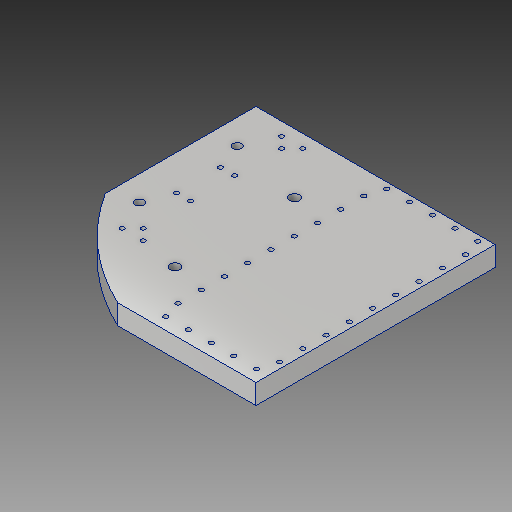
# Autodesk Inventor part: Base Plate Mk 2
Saved by Autodesk Inventor 2017 (Build 210142000, 142)
## iProperties
Created: 2016-12-06
Part Number: Base Plate Mk 2
Material: Aluminum 6061
Document SubType Name: Modeling
Designer: qupec
Density: 2.7 g/cm^3
Appearance: Aluminum - Flat
Mass: 732.131 g
Surface Area: 558.67 cm^2
Volume: 271.16 cm^3
Author: qupec
Autodesk Inventor part; units mm, degrees
ref_plane "YZ Plane" through (0, 0, 0) normal (1, 0, 0) x (0, 1, 0)
ref_plane "XZ Plane" through (0, 0, 0) normal (0, 1, 0) x (-1, 0, 0)
ref_plane "XY Plane" through (0, 0, 0) normal (0, 0, 1) x (1, 0, 0)
sketch "Sketch1" plane through (0, 0, 0) normal (0, 1, 0) x (-1, 0, 0)
  line L0 (76.2, 76.2) -> (-76.2, 76.2)
  line L1 (-76.2, 76.2) -> (-76.2, -76.2)
  line L2 (-76.2, -76.2) -> (76.2, -76.2)
  line L3 (76.2, -76.2) -> (76.2, 76.2)
  point P0 (0, 0)
  dimension "d0" = 152.4
  dimension "d1" = 152.4
  dimension "d2" = 76.2
  dimension "d3" = 76.2
  constraints: 8 end point, 2 parallel, 1 horizontal, 1 perpendicular
  measures "d0" distance of L2.end L0.start
  measures "d1" distance of L0.start L0.end
  measures "d2" distance from line of point (0, 0) L1
  measures "d3" distance from line of point (0, 0) L0
extrude "Extrusion1" add sketch "Sketch1" along normal blind 12.7
sketch "Sketch4" plane through (0, 12.7, 0) normal (0, 1, 0) x (1, 0, 0)
  circle A0 centre (69.85, 69.85) radius 3.175
  circle A1 centre (69.85, -69.85) radius 3.175
  circle A2 centre (-67.31, -52.07) radius 3.175
  line L0 (76.2, 76.2) -> (-76.2, 76.2) projected
  line L1 (76.2, -76.2) -> (76.2, 76.2) projected
  line L2 (-76.2, -76.2) -> (76.2, -76.2) projected
  line L3 (-76.2, 76.2) -> (-76.2, -76.2) projected
  circle A3 centre (-67.31, 52.07) radius 3.175
  point P0 (0, 0)
  dimension "d20" = 6.35
  dimension "d21" = 6.35
  dimension "d22" = 6.35
  dimension "d23" = 6.35
  dimension "d24" = 6.35
  dimension "d25" = 6.35
  dimension "d26" = 6.35
  dimension "d27" = 24.13
  dimension "d28" = 8.89
  dimension "d32" = 6.35
  dimension "d33" = 24.13
  dimension "d34" = 8.89
  constraints: 4 centre point
  measures "d20" diameter of A2
  measures "d21" diameter of A1
  measures "d22" diameter of A0
  measures "d23" distance from line of L0 A0.centre
  measures "d24" distance from line of L1 A0.centre
  measures "d25" distance from line of L1 A1.centre
  measures "d26" distance from line of L2 A1.centre
  measures "d27" distance from line of L2 A2.centre
  measures "d28" distance from line of L3 A2.centre
  measures "d32" diameter of A3
  measures "d33" distance from line of L0 A3.centre
  measures "d34" distance from line of L3 A3.centre
extrude "Extrusion6" [suppressed]
fillet "Fillet1" [suppressed]
sketch "Sketch7" plane through (0, 12.7, 0) normal (0, 1, 0) x (1, 0, 0)
  arc A0 (-76.2, -19.8745) -> (-11.9351, -76.2) centre (52.3545, 61.976) ccw
  line L0 (76.2, 76.2) -> (-76.2, 76.2) projected
  line L1 (76.2, -76.2) -> (76.2, 76.2) projected
  line L2 (-76.2, 76.2) -> (-76.2, -76.2) projected
  line L3 (-76.2, -76.2) -> (76.2, -76.2) projected
  line L4 (-76.2, 76.2) -> (-76.2, -76.2) projected
  arc A1 (-11.9351, -76.2) -> (-76.2, -19.8745) centre (52.3545, 61.976) ccw
  point P0 (0, 0)
  point P1 (76.2, -60.325)
  point P2 (73.025, -60.325)
  point P3 (73.025, 63.5)
  point P4 (73.025, 60.325)
  point P5 (-73.025, 63.5)
  point P6 (76.2, 60.325)
  point P7 (73.025, -63.5)
  point P8 (-76.2, 60.325)
  point P9 (-74.6455, -22.2663)
  dimension "d46" = 304.8
  dimension "d47" = 14.224
  dimension "d48" = 23.8455
  constraints: 5 point on circle, 2 centre point, 1 point on line, 3 other
  measures "d46" diameter of A0
  measures "d48" distance from line of L1 A0.centre
sketch "Sketch8" plane through (0, 12.7, 0) normal (0, 1, 0) x (1, 0, 0)
  circle A0 centre (-38.0726, -33.782) radius 1.4224 projected
  circle A1 centre (-44.8036, -27.051) radius 1.4224 projected
  circle A2 centre (-51.5346, -33.782) radius 1.4224 projected
  circle A3 centre (-51.5346, 67.818) radius 1.4224 projected
  circle A4 centre (-44.8036, 61.087) radius 1.4224 projected
  circle A5 centre (-38.0726, 67.818) radius 1.4224 projected
  circle A6 centre (-53.876, 3.1912) radius 1.4224 projected
  circle A7 centre (-53.876, 3.1912) radius 1.4224 projected
  circle A8 centre (-44.856, 3.1912) radius 1.4224 projected
  line L0 (-40.346, 0.6734) -> (-58.386, 0.6734) projected
  line L1 (-40.346, 5.7089) -> (-40.346, 0.6734) projected
  line L2 (-40.346, 5.7089) -> (-58.386, 5.7089) projected
  line L3 (-58.386, 0.6734) -> (-58.386, 5.7089) projected
  circle A9 centre (-53.876, 31.1756) radius 1.4224 projected
  circle A10 centre (-44.856, 31.1756) radius 1.4224 projected
  line L4 (-40.346, 28.6579) -> (-58.386, 28.6579) projected
  line L5 (-40.346, 33.6934) -> (-40.346, 28.6579) projected
  line L6 (-40.346, 33.6934) -> (-58.386, 33.6934) projected
  line L7 (-58.386, 28.6579) -> (-58.386, 33.6934) projected
  circle A11 centre (2.54, -39.6875) radius 3.175 construction
  circle A12 centre (2.54, 12.7127) radius 3.175 construction
  circle A13 centre (2.54, 65.1129) radius 3.175 construction
  circle A14 centre (68.58, 65.1129) radius 3.175 construction
  circle A15 centre (68.58, 12.7127) radius 3.175 construction
  circle A16 centre (68.58, -39.6875) radius 3.175 construction
extrude "Extrusion9" cut sketch "Sketch8" against normal through all contours A0 | A1 | A2 | A3 | A4 | A5 | A6 | A8 | A9 | A10
extrude "Extrusion11" cut sketch "Sketch7" against normal through all contours A0 L3 L2
sketch "Sketch10" plane through (0, 12.7, 0) normal (0, 1, 0) x (1, 0, 0)
  circle A0 centre (68.961, 72.39) radius 1.4732 projected
  arc A1 (-76.2, -19.8745) -> (-11.9351, -76.2) centre (52.3545, 61.976) ccw projected
  line L0 (-11.9351, -76.2) -> (76.2, -76.2) projected
  line L1 (76.2, -76.2) -> (76.2, 76.2) projected
  line L2 (76.2, 76.2) -> (-76.2, 76.2) projected
  line L3 (-76.2, 76.2) -> (-76.2, -19.8745) projected
  circle A2 centre (-53.876, 31.1756) radius 1.4224 projected
  circle A3 centre (-53.876, 3.1912) radius 1.4224 projected
  circle A4 centre (-44.8036, 61.087) radius 1.4224 projected
  circle A5 centre (-51.5346, -33.782) radius 1.4224 projected
  circle A6 centre (-38.0726, -33.782) radius 1.4224 projected
  circle A7 centre (-44.8036, -27.051) radius 1.4224 projected
  circle A8 centre (-51.5346, 67.818) radius 1.4224 projected
  circle A9 centre (-38.0726, 67.818) radius 1.4224 projected
  circle A10 centre (-44.856, 3.1912) radius 1.4224 projected
  circle A11 centre (-44.856, 31.1756) radius 1.4224 projected
  circle A12 centre (40.005, 72.39) radius 1.4732 projected
  circle A13 centre (54.483, 72.39) radius 1.4732 projected
  circle A14 centre (25.527, 72.39) radius 1.4732 projected
  circle A15 centre (11.049, 72.39) radius 1.4732 projected
  circle A16 centre (68.961, -68.58) radius 1.4732 projected
  circle A17 centre (54.483, -68.58) radius 1.4732 projected
  circle A18 centre (40.005, -68.58) radius 1.4732 projected
  circle A19 centre (25.527, -68.58) radius 1.4732 projected
  circle A20 centre (11.049, -68.58) radius 1.4732 projected
  point P0 (0, 0)
extrude "Extrusion13" cut sketch "Sketch10" against normal through all contours A0 | A12 | A13 | A14 | A15 | A16 | A17 | A18 | A19 | A20
sketch "Sketch11" plane through (0, 12.7, 0) normal (0, 1, 0) x (1, 0, 0)
  circle A0 centre (25.527, 72.39) radius 1.4732 projected
  circle A1 centre (54.483, 72.39) radius 1.4732 projected
  circle A2 centre (68.961, -68.58) radius 1.4732 projected
  circle A3 centre (40.005, -68.58) radius 1.4732 projected
  circle A4 centre (11.049, -68.58) radius 1.4732 projected
  circle A5 centre (7.62, -42.545) radius 1.4732 projected
  circle A6 centre (7.62, -12.9117) radius 1.4732 projected
  circle A7 centre (7.62, 16.7217) radius 1.4732 projected
  circle A8 centre (7.62, 46.355) radius 1.4732 projected
  circle A9 centre (72.39, 61.1717) radius 1.4732 projected
  circle A10 centre (72.39, 31.5383) radius 1.4732 projected
  circle A11 centre (72.39, 1.905) radius 1.4732 projected
  circle A12 centre (72.39, -27.7283) radius 1.4732 projected
  circle A13 centre (72.39, -57.3617) radius 1.4732 projected
  circle A14 centre (72.39, -42.545) radius 1.4732 projected
  circle A15 centre (72.39, -12.9117) radius 1.4732 projected
  circle A16 centre (72.39, 16.7217) radius 1.4732 projected
  circle A17 centre (72.39, 46.355) radius 1.4732 projected
  circle A18 centre (7.62, 61.1717) radius 1.4732 projected
  circle A19 centre (7.62, 31.5383) radius 1.4732 projected
  circle A20 centre (7.62, 1.905) radius 1.4732 projected
  circle A21 centre (7.62, -27.7283) radius 1.4732 projected
  circle A22 centre (7.62, -57.3617) radius 1.4732 projected
  circle A23 centre (25.527, -68.58) radius 1.4732 projected
  circle A24 centre (54.483, -68.58) radius 1.4732 projected
  circle A25 centre (68.961, 72.39) radius 1.4732 projected
  circle A26 centre (40.005, 72.39) radius 1.4732 projected
  circle A27 centre (11.049, 72.39) radius 1.4732 projected
  line L0 (6.985, -72.39) -> (73.025, -72.39) projected
  line L1 (76.2, -69.215) -> (76.2, 73.025) projected
  line L2 (73.025, 76.2) -> (6.985, 76.2) projected
  line L3 (3.81, 73.025) -> (3.81, -69.215) projected
  arc A28 (65.405, 62.23) -> (62.23, 65.405) centre (62.23, 62.23) ccw projected
  line L4 (65.405, -58.42) -> (65.405, 62.23) projected
  arc A29 (62.23, -61.595) -> (65.405, -58.42) centre (62.23, -58.42) ccw projected
  line L5 (17.78, -61.595) -> (62.23, -61.595) projected
  arc A30 (14.605, -58.42) -> (17.78, -61.595) centre (17.78, -58.42) ccw projected
  line L6 (14.605, 62.23) -> (14.605, -58.42) projected
  arc A31 (17.78, 65.405) -> (14.605, 62.23) centre (17.78, 62.23) ccw projected
  line L7 (62.23, 65.405) -> (17.78, 65.405) projected
  arc A32 (76.2, 73.025) -> (73.025, 76.2) centre (73.025, 73.025) ccw projected
  arc A33 (6.985, 76.2) -> (3.81, 73.025) centre (6.985, 73.025) ccw projected
  arc A34 (3.81, -69.215) -> (6.985, -72.39) centre (6.985, -69.215) ccw projected
  arc A35 (73.025, -72.39) -> (76.2, -69.215) centre (73.025, -69.215) ccw projected
  point P0 (0, 0)
extrude "Extrusion14" cut sketch "Sketch11" against normal through all contours A5 | A6 | A7 | A8 | A9 | A10 | A11 | A12 | A13 | A14 | A15 | A16 | A17 | A18 | A19 | A20 | A21 | A22 | A25
sketch "Sketch12" plane through (0, 12.7, 0) normal (0, 1, 0) x (1, 0, 0)
  line L0 (-76.2, 76.2) -> (-76.2, -19.8745) projected
  line L1 (76.2, 76.2) -> (-76.2, 76.2) projected
  circle A0 centre (-53.876, 31.1756) radius 1.4224 projected
  circle A1 centre (-53.876, 3.1912) radius 1.4224 projected
  line L2 (-53.876, 17.1834) -> (-44.4208, 17.1834) construction
  point P0 (0, 0)
  point P1 (-60.325, -13.9316)
  point P2 (-60.325, 48.2984)
  dimension "d63" = 15.875
  dimension "d64" = 15.875
  dimension "d75" = 13.9922
  dimension "d76" = 27.9845
  dimension "d77" = 31.115
  dimension "d78" = 31.115
  constraints: 2 end point, 1 horizontal
  measures "d63" distance from line of L0 point (-60.325, 48.298)
  measures "d64" distance from line of L0 point (-60.325, -13.932)
  measures "d75" distance from line of A1.centre L2
  measures "d76" distance of A0.centre A1.centre
  measures "d77" distance from line of L2 point (-60.325, -13.932)
  measures "d78" distance from line of L2 point (-60.325, 48.298)
hole "Hole1" at (-60.325, 12.7, 13.9316) at (-60.325, 12.7, -48.2984) direction (0, -1, 0) diameter 5.588 depth 25.4 tip angle 118
sketch "Sketch14" plane through (0, 0, 0) normal (0, -1, 0) x (1, 0, 0)
  line L0 (76.2, -76.2) -> (-76.2, -76.2) projected
  line L1 (-11.9351, 76.2) -> (76.2, 76.2) projected
  circle A0 centre (11.049, -72.39) radius 1.4732 projected
  circle A1 centre (-38.0726, -67.818) radius 1.4224 projected
  point P0 (0, 0)
  point P1 (-13.5118, 38.1)
  point P2 (-13.5118, -38.1)
  dimension "d79" = 38.1
  dimension "d80" = 152.4
  dimension "d81" = 38.1
  dimension "d82" = 49.1217
  dimension "d83" = 24.5608
  dimension "d84" = 24.5608
  measures "d79" vertical distance of point (0, 0) point (-13.512, 38.1)
  measures "d80" distance between parallel lines of L0 L1
  measures "d81" vertical distance of point (-13.512, -38.1) point (0, 0)
  measures "d82" horizontal distance of A0.centre A1.centre
  measures "d83" horizontal distance of A1.centre point (-13.512, -38.1)
  measures "d84" horizontal distance of A1.centre point (-13.512, 38.1)
hole "Hole2" at (-13.5118, 0, 38.1) at (-13.5118, 0, -38.1) direction (0, 1, 0) diameter 6.35 depth 25.4 tip angle 118
sketch "Sketch15" plane through (0, 0, 0) normal (0, -1, 0) x (1, 0, 0)
  circle A0 centre (-13.5118, 38.1) radius 3.175 projected
  circle A1 centre (-13.5118, -38.1) radius 3.175 projected
  circle A2 centre (72.39, -31.5383) radius 1.4732 projected
  circle A3 centre (7.62, -31.5383) radius 1.4732 projected
  circle A4 centre (7.62, 42.545) radius 1.4732 projected
  point P0 (0, 0)
  point P1 (40.005, -38.1)
  point P2 (40.005, 38.1)
  dimension "d92" = 38.1
  dimension "d93" = 38.1
  dimension "d94" = 38.1
  dimension "d95" = 38.1
  dimension "d96" = 64.77
  dimension "d97" = 32.385
  dimension "d98" = 32.385
  measures "d92" vertical distance of point (0, 0) point (40.005, 38.1)
  measures "d93" vertical distance of point (0, 0) A0.centre
  measures "d94" vertical distance of point (0, 0) A1.centre
  measures "d95" vertical distance of point (40.005, -38.1) point (0, 0)
  measures "d96" distance between centres of A2 A3
  measures "d97" horizontal distance of A3.centre point (40.005, -38.1)
  measures "d98" horizontal distance of point (40.005, 38.1) A4.centre
hole "Hole3" at (40.005, 0, -38.1) at (40.005, 0, 38.1) direction (0, 1, 0) diameter 6.35 depth 9.525
thread "Thread1" size "1/4-20 UNC" class "2B" standard "ANSI Unified Screw Threads" full length
thread "Thread2" size "1/4-20 UNC" class "2B" standard "ANSI Unified Screw Threads" full length
equation "\"d2\" = 0.5 * d1"
equation "\"d3\" = 0.5 * d0"
equation "\"d21\" = d20"
equation "\"d22\" = d20"
equation "\"d24\" = d23"
equation "\"d25\" = d24"
equation "\"d26\" = d23"
equation "\"d32\" = d20"
equation "\"d33\" = d27"
equation "\"d34\" = d28"
equation "\"d63\" = d64"
equation "\"d75\" = 0.5 * d76"
equation "\"d78\" = d77"
equation "\"d83\" = 0.5 * d82"
equation "\"d84\" = d83"
equation "\"d92\" = d93"
equation "\"d95\" = d94"
equation "\"d97\" = 0.5 * d96"
equation "\"d98\" = d97"
body "Solid1"
